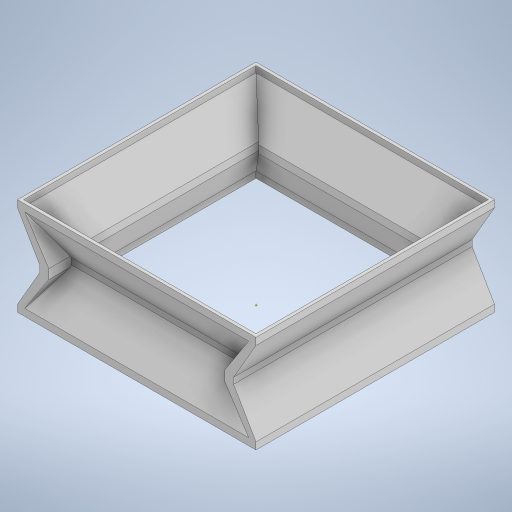
# Autodesk Inventor part: 사각형 OV-PAM 5패턴 층 한개
Saved by Autodesk Inventor 2024 (Build 280153000, 153)
## iProperties
Created: 2023-06-16
Part Number: 사각형 OV-PAM 5패턴 층 한개
Material: 일반
Document SubType Name: Modeling
Designer: jsw
Density: 1 g/cm^3
Appearance: 기본값
Author: jsw
Autodesk Inventor part; units mm, degrees
ref_plane "YZ Plane" through (0, 0, 0) normal (1, 0, 0) x (0, 1, 0)
ref_plane "XZ Plane" through (0, 0, 0) normal (0, 1, 0) x (-1, 0, 0)
ref_plane "XY Plane" through (0, 0, 0) normal (0, 0, 1) x (1, 0, 0)
sketch "스케치1" plane through (0, 0, 0) normal (0, 1, 0) x (-1, 0, 0)
  line L0 (0, 0) -> (-60, 0)
  line L1 (-60, 0) -> (-60, -60)
  line L2 (-60, -60) -> (0, -60)
  line L3 (0, -60) -> (0, 0)
  dimension "d0" = 60
  dimension "d1" = 60
  constraints: 8 end point, 2 parallel, 1 horizontal, 1 perpendicular
  measures "d0" distance of L2.end L1.end
  measures "d1" distance of L1.end L0.end
extrude "돌출1" add sketch "스케치1" along normal blind 10
ref_plane "작업 평면1" through (0, 0, 0) normal (0, 0.5, 0.8660254) x (1, 0, 0)
sketch "스케치2" plane through (0, 0, 0) normal (0, 0, 1) x (1, 0, 0)
  line L0 (60, 0) -> (0, 0) projected
  line L1 (0, 0) -> (6.4941, 10)
  line L2 (60, 10) -> (0, 10) projected
  line L3 (60, 0) -> (53.5059, 10)
  line L4 (6.4941, 10) -> (53.5059, 10)
  line L5 (60, 0) -> (0, 0)
  point P0 (53.5059, 10)
  dimension "d6" = 57
  dimension "d7" = 57
  constraints: 8 end point, 2 collinear, 1 point on line
  measures "d6" angle of L1 L2
  measures "d7" angle of L2 L3
extrude "돌출2" cut sketch "스케치2" against normal up to surface surface through (0, 0, 0) normal (0, 0.5, 0.8660254)
ref_plane "작업 평면2" through (60, 0, 0) normal (0.8660254, 0.5, 0) x (0, 0, -1)
sketch "스케치3" plane through (60, 0, -60) normal (1, 0, 0) x (0, 0, -1)
  line L0 (0, 10) -> (-60, 10) projected
  line L1 (-60, 10) -> (0, 10)
  line L2 (0, 10) -> (0, 0)
  line L3 (0, 0) -> (-60, 0)
  line L4 (-60, 0) -> (-60, 10)
  line L5 (-60, 0) -> (-65.7735, 10)
  line L6 (-65.7735, 10) -> (-60, 10)
  line L7 (0, 0) -> (5.7735, 10)
  line L8 (5.7735, 10) -> (0, 10)
  dimension "d11" = 120
  dimension "d12" = 120
  constraints: 16 end point, 2 collinear, 2 parallel, 1 horizontal, 1 perpendicular, 1 point on line
  measures "d11" angle of L5 L3
  measures "d12" angle of L3 L7
extrude "돌출3" cut sketch "스케치3" against normal up to surface surface through (60, 0, 0) normal (0.8660254, 0.5, 0)
pattern_circular "원형 패턴1" count 2 over 360 about axis through (30, 0, -30) along (0, -1, 0) of "돌출3", "돌출2"
ref_plane "작업 평면3" through (0, 11, 0) normal (0, 1, 0) x (1, 0, 0)
mirror "미러1" about plane through (0, 11, 0) normal (0, 1, 0) of "돌출3", "돌출2", "돌출1", "원형 패턴1"
sketch "스케치4" plane through (0, 11, 0) normal (0, 1, 0) x (1, 0, 0)
  line L0 (5.7735, 60) -> (5.7735, 0) projected
  line L1 (5.7735, 0) -> (6.4941, 0) projected
  line L2 (6.4941, 0) -> (6.4941, 5.7735) projected
  line L3 (6.4941, 5.7735) -> (53.5059, 5.7735) projected
  line L4 (53.5059, 5.7735) -> (53.5059, 0) projected
  line L5 (53.5059, 0) -> (54.2265, 0) projected
  line L6 (54.2265, 0) -> (54.2265, 60) projected
  line L7 (54.2265, 60) -> (53.5059, 60) projected
  line L8 (53.5059, 60) -> (53.5059, 54.2265) projected
  line L9 (53.5059, 54.2265) -> (6.4941, 54.2265) projected
  line L10 (6.4941, 54.2265) -> (6.4941, 60) projected
  line L11 (6.4941, 60) -> (5.7735, 60) projected
  point P0 (0, 0)
extrude "돌출4" add sketch "스케치4" along normal mid plane 2
sketch "스케치5" plane through (0, 22, -60) normal (0, 1, 0) x (1, 0, 0)
  line L0 (0, -60) -> (0, 0) projected
  line L1 (0, 0) -> (60, 0) projected
  line L2 (60, 0) -> (60, -60) projected
  line L3 (60, -60) -> (0, -60) projected
extrude "돌출5" add sketch "스케치5" along normal blind 1.6
mirror "미러2" about plane through (0, 11, 0) normal (0, 1, 0) of "돌출5"
shell "쉘2" thickness 0.8 outward yes removed faces 2 at (40, 23.6, -20) at (40, -1.6, -20)
